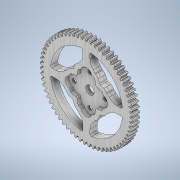
# Autodesk Inventor part: アーム 2段目ギア 大ギア 64
Saved by Autodesk Inventor 2020.2 (Build 242310000, 310)
## iProperties
Created: 2020-05-01
Part Number: アーム 2段目ギア 大ギア 64
Material: アルミニウム 7075
Document SubType Name: Modeling
Designer: mozar
Density: 2.81 g/cm^3
Appearance: サテン - ブラシ仕上げ 重厚
Author: mozar
Autodesk Inventor part; units mm, degrees
(part 1 of 5)
ref_plane "YZ Plane" through (0, 0, 0) normal (1, 0, 0) x (0, 1, 0)
ref_plane "XZ Plane" through (0, 0, 0) normal (0, 1, 0) x (-1, 0, 0)
ref_plane "XY Plane" through (0, 0, 0) normal (0, 0, 1) x (1, 0, 0)
sketch "スケッチ1" plane through (0, 0, 0) normal (0, 0, 1) x (1, 0, 0)
  arc A0 (149.0434, 136.3017) -> (148.894, 135.7475) centre (156.2837, 134.0527) ccw
  arc A1 (149.3046, 137.0392) -> (149.0434, 136.3017) centre (158.5049, 133.3653) ccw
  arc A2 (149.7251, 137.9773) -> (149.3046, 137.0392) centre (160.7701, 132.4624) ccw
  arc A3 (145.9727, 136.2043) -> (145.8783, 135.638) centre (153.3985, 134.6758) ccw
  arc A4 (146.1603, 136.9638) -> (145.9727, 136.2043) centre (155.6764, 134.2093) ccw
  arc A5 (146.4869, 137.9385) -> (146.1603, 136.9638) centre (158.0193, 133.5328) ccw
  arc A6 (142.9263, 135.8063) -> (142.8879, 135.2335) centre (150.4662, 135.013) ccw
  arc A7 (143.0386, 136.5805) -> (142.9263, 135.8063) centre (152.7789, 134.7721) ccw
  arc A8 (143.2681, 137.5826) -> (143.0386, 136.5805) centre (155.1767, 134.3285) ccw
  arc A9 (139.9336, 135.1116) -> (139.9515, 134.5379) centre (147.515, 135.0612) ccw
  arc A10 (139.9695, 135.8932) -> (139.9336, 135.1116) centre (149.8401, 135.0481) ccw
  arc A11 (140.0996, 136.9129) -> (139.9695, 135.8932) centre (152.2699, 134.8417) ccw
  arc A12 (137.0234, 134.127) -> (137.0974, 133.5577) centre (144.5732, 134.8199) ccw
  arc A13 (136.9825, 134.9083) -> (137.0234, 134.127) centre (146.8884, 135.0348) ccw
  arc A14 (137.012, 135.9358) -> (136.9825, 134.9083) centre (149.3267, 135.0675) ccw
  arc A15 (134.2237, 132.8618) -> (134.3532, 132.3026) centre (141.6692, 134.2914) ccw
  arc A16 (134.1064, 133.6353) -> (134.2237, 132.8618) centre (143.9522, 134.7322) ccw
  arc A17 (134.0351, 134.6609) -> (134.1064, 133.6353) centre (146.3756, 135.0037) ccw
  arc A18 (131.5615, 131.3283) -> (131.7452, 130.7845) centre (138.8311, 133.4809) ccw
  arc A19 (131.369, 132.0866) -> (131.5615, 131.3283) centre (141.0599, 134.1433) ccw
  arc A20 (131.1975, 133.1002) -> (131.369, 132.0866) centre (143.445, 134.651) ccw
  arc A21 (129.0624, 129.5413) -> (129.2985, 129.018) centre (136.086, 132.396) ccw
  arc A22 (128.7965, 130.2771) -> (129.0624, 129.5413) centre (138.2392, 133.2737) ccw
  arc A23 (128.5265, 131.269) -> (128.7965, 130.2771) centre (140.563, 134.0128) ccw
  arc A24 (126.7505, 127.5179) -> (127.0368, 127.0203) centre (133.4605, 131.0473) ccw
  arc A25 (126.4138, 128.2241) -> (126.7505, 127.5179) centre (135.5173, 132.1318) ccw
  arc A26 (126.0479, 129.1847) -> (126.4138, 128.2241) centre (137.7575, 133.0951) ccw
  arc A27 (124.6481, 125.2777) -> (124.9818, 124.8105) centre (130.9799, 129.4477) ccw
  arc A28 (124.2438, 125.9474) -> (124.6481, 125.2777) centre (132.9204, 130.7286) ccw
  arc A29 (123.7855, 126.8676) -> (124.2438, 125.9474) centre (135.0554, 131.9069) ccw
  arc A30 (122.7754, 122.8421) -> (123.1533, 122.41) centre (128.6679, 127.6127) ccw
  arc A31 (122.3074, 123.469) -> (122.7754, 122.8421) centre (130.4736, 129.0776) ccw
  arc A32 (121.7611, 124.3398) -> (122.3074, 123.469) centre (132.4828, 130.4595) ccw
  arc A33 (121.1505, 120.2348) -> (121.5689, 119.8417) centre (126.547, 125.56) ccw
  arc A34 (120.6232, 120.8128) -> (121.1505, 120.2348) centre (128.2004, 127.1948) ccw
  arc A35 (119.9942, 121.6258) -> (120.6232, 120.8128) centre (130.0645, 128.767) ccw
  arc A36 (119.7889, 117.4807) -> (120.2438, 117.1305) centre (124.6375, 123.3092) ccw
  arc A37 (119.2076, 118.0042) -> (119.7889, 117.4807) centre (126.1226, 125.0982) ccw
  arc A38 (118.5018, 118.7517) -> (119.2076, 118.0042) centre (127.8237, 126.8455) ccw
  arc A39 (118.7038, 114.6064) -> (119.1909, 114.3025) centre (122.9578, 120.8821) ccw
  arc A40 (118.074, 115.0704) -> (118.7038, 114.6064) centre (124.2604, 122.8081) ccw
  arc A41 (117.2984, 115.7452) -> (118.074, 115.0704) centre (125.782, 124.7137) ccw
  arc A42 (117.9057, 111.6396) -> (118.4202, 111.3849) centre (121.524, 118.302) ccw
  arc A43 (117.2334, 112.0397) -> (117.9057, 111.6396) centre (122.6316, 120.3464) ccw
  arc A44 (116.3954, 112.6351) -> (117.2334, 112.0397) centre (123.9591, 122.392) ccw
  arc A45 (117.4022, 108.6089) -> (117.9392, 108.4058) centre (120.3501, 115.5939) ccw
  arc A46 (116.6939, 108.9411) -> (117.4022, 108.6089) centre (121.252, 117.737) ccw
  arc A47 (115.8016, 109.4516) -> (116.6939, 108.9411) centre (122.3726, 119.9028) ccw
  arc A48 (117.1983, 105.5434) -> (117.7525, 105.394) centre (119.4473, 112.7837) ccw
  arc A49 (116.4608, 105.8046) -> (117.1983, 105.5434) centre (120.1347, 115.0049) ccw
  arc A50 (115.5227, 106.2251) -> (116.4608, 105.8046) centre (121.0376, 117.2701) ccw
  arc A51 (117.2957, 102.4727) -> (117.862, 102.3783) centre (118.8242, 109.8985) ccw
  arc A52 (116.5362, 102.6603) -> (117.2957, 102.4727) centre (119.2907, 112.1764) ccw
  arc A53 (115.5615, 102.9869) -> (116.5362, 102.6603) centre (119.9672, 114.5193) ccw
  arc A54 (117.6937, 99.4263) -> (118.2665, 99.3879) centre (118.487, 106.9662) ccw
  arc A55 (116.9195, 99.5386) -> (117.6937, 99.4263) centre (118.7279, 109.2789) ccw
  arc A56 (115.9174, 99.7681) -> (116.9195, 99.5386) centre (119.1715, 111.6767) ccw
  arc A57 (118.3884, 96.4336) -> (118.9621, 96.4515) centre (118.4388, 104.015) ccw
  arc A58 (117.6068, 96.4695) -> (118.3884, 96.4336) centre (118.4519, 106.3401) ccw
  arc A59 (116.5871, 96.5996) -> (117.6068, 96.4695) centre (118.6583, 108.7699) ccw
  arc A60 (119.373, 93.5234) -> (119.9423, 93.5974) centre (118.6801, 101.0732) ccw
  arc A61 (118.5917, 93.4825) -> (119.373, 93.5234) centre (118.4652, 103.3884) ccw
  arc A62 (117.5642, 93.512) -> (118.5917, 93.4825) centre (118.4325, 105.8267) ccw
  arc A63 (120.6382, 90.7237) -> (121.1974, 90.8532) centre (119.2086, 98.1692) ccw
  arc A64 (119.8647, 90.6064) -> (120.6382, 90.7237) centre (118.7678, 100.4522) ccw
  arc A65 (118.8391, 90.5351) -> (119.8647, 90.6064) centre (118.4963, 102.8756) ccw
  arc A66 (122.1717, 88.0615) -> (122.7155, 88.2452) centre (120.0191, 95.3311) ccw
  arc A67 (121.4134, 87.869) -> (122.1717, 88.0615) centre (119.3567, 97.5599) ccw
  arc A68 (120.3998, 87.6975) -> (121.4134, 87.869) centre (118.849, 99.945) ccw
  arc A69 (123.9587, 85.5624) -> (124.482, 85.7985) centre (121.104, 92.586) ccw
  arc A70 (123.2229, 85.2965) -> (123.9587, 85.5624) centre (120.2263, 94.7392) ccw
  arc A71 (122.231, 85.0265) -> (123.2229, 85.2965) centre (119.4872, 97.063) ccw
  arc A72 (125.9821, 83.2505) -> (126.4797, 83.5368) centre (122.4527, 89.9605) ccw
  arc A73 (125.2759, 82.9138) -> (125.9821, 83.2505) centre (121.3682, 92.0173) ccw
  arc A74 (124.3153, 82.5479) -> (125.2759, 82.9138) centre (120.4049, 94.2575) ccw
  arc A75 (128.2223, 81.1481) -> (128.6895, 81.4818) centre (124.0523, 87.4799) ccw
  arc A76 (127.5526, 80.7438) -> (128.2223, 81.1481) centre (122.7714, 89.4204) ccw
  arc A77 (126.6324, 80.2855) -> (127.5526, 80.7438) centre (121.5931, 91.5554) ccw
  arc A78 (130.6579, 79.2754) -> (131.09, 79.6533) centre (125.8873, 85.1679) ccw
  arc A79 (130.031, 78.8074) -> (130.6579, 79.2754) centre (124.4224, 86.9736) ccw
  arc A80 (129.1602, 78.2611) -> (130.031, 78.8074) centre (123.0405, 88.9828) ccw
  arc A81 (133.2652, 77.6505) -> (133.6583, 78.0689) centre (127.94, 83.047) ccw
  arc A82 (132.6872, 77.1232) -> (133.2652, 77.6505) centre (126.3052, 84.7004) ccw
  arc A83 (131.8742, 76.4942) -> (132.6872, 77.1232) centre (124.733, 86.5645) ccw
  arc A84 (136.0193, 76.2889) -> (136.3695, 76.7438) centre (130.1908, 81.1375) ccw
  arc A85 (135.4958, 75.7076) -> (136.0193, 76.2889) centre (128.4018, 82.6226) ccw
  arc A86 (134.7483, 75.0018) -> (135.4958, 75.7076) centre (126.6545, 84.3237) ccw
  arc A87 (138.8936, 75.2038) -> (139.1975, 75.6909) centre (132.6179, 79.4578) ccw
  arc A88 (138.4296, 74.574) -> (138.8936, 75.2038) centre (130.6919, 80.7604) ccw
  arc A89 (137.7548, 73.7984) -> (138.4296, 74.574) centre (128.7863, 82.282) ccw
  arc A90 (141.8604, 74.4057) -> (142.1151, 74.9202) centre (135.198, 78.024) ccw
  arc A91 (141.4603, 73.7334) -> (141.8604, 74.4057) centre (133.1536, 79.1316) ccw
  arc A92 (140.8649, 72.8954) -> (141.4603, 73.7334) centre (131.108, 80.4591) ccw
  arc A93 (144.8911, 73.9022) -> (145.0942, 74.4392) centre (137.9061, 76.8501) ccw
  arc A94 (144.5589, 73.1939) -> (144.8911, 73.9022) centre (135.763, 77.752) ccw
  arc A95 (144.0484, 72.3016) -> (144.5589, 73.1939) centre (133.5972, 78.8726) ccw
  arc A96 (147.9566, 73.6983) -> (148.106, 74.2525) centre (140.7163, 75.9473) ccw
  arc A97 (147.6954, 72.9608) -> (147.9566, 73.6983) centre (138.4951, 76.6347) ccw
  arc A98 (147.2749, 72.0227) -> (147.6954, 72.9608) centre (136.2299, 77.5376) ccw
  arc A99 (151.0273, 73.7957) -> (151.1217, 74.362) centre (143.6015, 75.3242) ccw
  arc A100 (150.8397, 73.0362) -> (151.0273, 73.7957) centre (141.3236, 75.7907) ccw
  arc A101 (150.5131, 72.0615) -> (150.8397, 73.0362) centre (138.9807, 76.4672) ccw
  arc A102 (154.0737, 74.1937) -> (154.1121, 74.7665) centre (146.5338, 74.987) ccw
  arc A103 (153.9614, 73.4195) -> (154.0737, 74.1937) centre (144.2211, 75.2279) ccw
  arc A104 (153.7319, 72.4174) -> (153.9614, 73.4195) centre (141.8233, 75.6715) ccw
  arc A105 (157.0664, 74.8884) -> (157.0485, 75.4621) centre (149.485, 74.9388) ccw
  arc A106 (157.0305, 74.1068) -> (157.0664, 74.8884) centre (147.1599, 74.9519) ccw
  arc A107 (156.9004, 73.0871) -> (157.0305, 74.1068) centre (144.7301, 75.1583) ccw
  arc A108 (159.9766, 75.873) -> (159.9026, 76.4423) centre (152.4268, 75.1801) ccw
  arc A109 (160.0175, 75.0917) -> (159.9766, 75.873) centre (150.1116, 74.9652) ccw
  arc A110 (159.988, 74.0642) -> (160.0175, 75.0917) centre (147.6733, 74.9325) ccw
  arc A111 (162.7763, 77.1382) -> (162.6468, 77.6974) centre (155.3308, 75.7086) ccw
  arc A112 (162.8936, 76.3647) -> (162.7763, 77.1382) centre (153.0478, 75.2678) ccw
  arc A113 (162.9649, 75.3391) -> (162.8936, 76.3647) centre (150.6244, 74.9963) ccw
  arc A114 (165.4385, 78.6717) -> (165.2548, 79.2155) centre (158.1689, 76.5191) ccw
  arc A115 (165.631, 77.9134) -> (165.4385, 78.6717) centre (155.9401, 75.8567) ccw
  arc A116 (165.8025, 76.8998) -> (165.631, 77.9134) centre (153.555, 75.349) ccw
  arc A117 (167.9376, 80.4587) -> (167.7015, 80.982) centre (160.914, 77.604) ccw
  arc A118 (168.2035, 79.7229) -> (167.9376, 80.4587) centre (158.7608, 76.7263) ccw
  arc A119 (168.4735, 78.731) -> (168.2035, 79.7229) centre (156.437, 75.9872) ccw
  arc A120 (170.2495, 82.4821) -> (169.9632, 82.9797) centre (163.5395, 78.9527) ccw
  arc A121 (170.5862, 81.7759) -> (170.2495, 82.4821) centre (161.4827, 77.8682) ccw
  arc A122 (170.9521, 80.8153) -> (170.5862, 81.7759) centre (159.2425, 76.9049) ccw
  arc A123 (172.3519, 84.7223) -> (172.0182, 85.1895) centre (166.0201, 80.5523) ccw
  arc A124 (172.7562, 84.0526) -> (172.3519, 84.7223) centre (164.0796, 79.2714) ccw
  arc A125 (173.2145, 83.1324) -> (172.7562, 84.0526) centre (161.9446, 78.0931) ccw
  arc A126 (174.2246, 87.1579) -> (173.8467, 87.59) centre (168.3321, 82.3873) ccw
  arc A127 (174.6926, 86.531) -> (174.2246, 87.1579) centre (166.5264, 80.9224) ccw
  arc A128 (175.2389, 85.6602) -> (174.6926, 86.531) centre (164.5172, 79.5405) ccw
  arc A129 (175.8495, 89.7652) -> (175.4311, 90.1583) centre (170.453, 84.44) ccw
  arc A130 (176.3768, 89.1872) -> (175.8495, 89.7652) centre (168.7996, 82.8052) ccw
  arc A131 (177.0058, 88.3742) -> (176.3768, 89.1872) centre (166.9355, 81.233) ccw
  arc A132 (177.2111, 92.5193) -> (176.7562, 92.8695) centre (172.3625, 86.6908) ccw
  arc A133 (177.7924, 91.9958) -> (177.2111, 92.5193) centre (170.8774, 84.9018) ccw
  arc A134 (178.4982, 91.2483) -> (177.7924, 91.9958) centre (169.1763, 83.1545) ccw
  arc A135 (178.2962, 95.3936) -> (177.8091, 95.6975) centre (174.0422, 89.1179) ccw
  arc A136 (178.926, 94.9296) -> (178.2962, 95.3936) centre (172.7396, 87.1919) ccw
  arc A137 (179.7016, 94.2548) -> (178.926, 94.9296) centre (171.218, 85.2863) ccw
  arc A138 (179.0943, 98.3604) -> (178.5798, 98.6151) centre (175.476, 91.698) ccw
  arc A139 (179.7666, 97.9603) -> (179.0943, 98.3604) centre (174.3684, 89.6536) ccw
  arc A140 (180.6046, 97.3649) -> (179.7666, 97.9603) centre (173.0409, 87.608) ccw
  arc A141 (179.5978, 101.3911) -> (179.0608, 101.5942) centre (176.6499, 94.4061) ccw
  arc A142 (180.3061, 101.0589) -> (179.5978, 101.3911) centre (175.748, 92.263) ccw
  arc A143 (181.1984, 100.5484) -> (180.3061, 101.0589) centre (174.6274, 90.0972) ccw
  arc A144 (179.8017, 104.4566) -> (179.2475, 104.606) centre (177.5527, 97.2163) ccw
  arc A145 (180.5392, 104.1954) -> (179.8017, 104.4566) centre (176.8653, 94.9951) ccw
  arc A146 (181.4773, 103.7749) -> (180.5392, 104.1954) centre (175.9624, 92.7299) ccw
  arc A147 (179.7043, 107.5273) -> (179.138, 107.6217) centre (178.1758, 100.1015) ccw
  arc A148 (180.4638, 107.3397) -> (179.7043, 107.5273) centre (177.7093, 97.8236) ccw
  arc A149 (181.4385, 107.0131) -> (180.4638, 107.3397) centre (177.0328, 95.4807) ccw
  arc A150 (179.3063, 110.5737) -> (178.7335, 110.6121) centre (178.513, 103.0338) ccw
  arc A151 (180.0805, 110.4614) -> (179.3063, 110.5737) centre (178.2721, 100.7211) ccw
  arc A152 (181.0826, 110.2319) -> (180.0805, 110.4614) centre (177.8285, 98.3233) ccw
  arc A153 (178.6116, 113.5664) -> (178.0379, 113.5485) centre (178.5612, 105.985) ccw
  arc A154 (179.3932, 113.5305) -> (178.6116, 113.5664) centre (178.5481, 103.6599) ccw
  arc A155 (180.4129, 113.4004) -> (179.3932, 113.5305) centre (178.3417, 101.2301) ccw
  arc A156 (177.627, 116.4766) -> (177.0577, 116.4026) centre (178.3199, 108.9268) ccw
  arc A157 (178.4083, 116.5175) -> (177.627, 116.4766) centre (178.5348, 106.6116) ccw
  arc A158 (179.4358, 116.488) -> (178.4083, 116.5175) centre (178.5675, 104.1733) ccw
  arc A159 (176.3618, 119.2763) -> (175.8026, 119.1468) centre (177.7914, 111.8308) ccw
  arc A160 (177.1353, 119.3936) -> (176.3618, 119.2763) centre (178.2322, 109.5478) ccw
  arc A161 (178.1609, 119.4649) -> (177.1353, 119.3936) centre (178.5037, 107.1244) ccw
  arc A162 (174.8283, 121.9385) -> (174.2845, 121.7548) centre (176.9809, 114.6689) ccw
  arc A163 (175.5866, 122.131) -> (174.8283, 121.9385) centre (177.6433, 112.4401) ccw
  arc A164 (176.6002, 122.3025) -> (175.5866, 122.131) centre (178.151, 110.055) ccw
  arc A165 (173.0413, 124.4376) -> (172.518, 124.2015) centre (175.896, 117.414) ccw
  arc A166 (173.7771, 124.7035) -> (173.0413, 124.4376) centre (176.7737, 115.2608) ccw
  arc A167 (174.769, 124.9735) -> (173.7771, 124.7035) centre (177.5128, 112.937) ccw
  arc A168 (171.0179, 126.7495) -> (170.5203, 126.4632) centre (174.5473, 120.0395) ccw
  arc A169 (171.7241, 127.0862) -> (171.0179, 126.7495) centre (175.6318, 117.9827) ccw
  arc A170 (172.6847, 127.4521) -> (171.7241, 127.0862) centre (176.5951, 115.7425) ccw
  arc A171 (168.7777, 128.8519) -> (168.3105, 128.5182) centre (172.9477, 122.5201) ccw
  arc A172 (169.4474, 129.2562) -> (168.7777, 128.8519) centre (174.2286, 120.5796) ccw
  arc A173 (170.3676, 129.7145) -> (169.4474, 129.2562) centre (175.4069, 118.4446) ccw
  arc A174 (166.3421, 130.7246) -> (165.91, 130.3467) centre (171.1127, 124.8321) ccw
  arc A175 (166.969, 131.1926) -> (166.3421, 130.7246) centre (172.5776, 123.0264) ccw
  arc A176 (167.8398, 131.7389) -> (166.969, 131.1926) centre (173.9595, 121.0172) ccw
  arc A177 (163.7348, 132.3495) -> (163.3417, 131.9311) centre (169.06, 126.953) ccw
  arc A178 (164.3128, 132.8768) -> (163.7348, 132.3495) centre (170.6948, 125.2996) ccw
  arc A179 (165.1258, 133.5058) -> (164.3128, 132.8768) centre (172.267, 123.4355) ccw
  arc A180 (160.9807, 133.7111) -> (160.6305, 133.2562) centre (166.8092, 128.8625) ccw
  arc A181 (161.5042, 134.2924) -> (160.9807, 133.7111) centre (168.5982, 127.3774) ccw
  arc A182 (162.2517, 134.9982) -> (161.5042, 134.2924) centre (170.3455, 125.6763) ccw
  arc A183 (158.1064, 134.7962) -> (157.8025, 134.3091) centre (164.3821, 130.5422) ccw
  arc A184 (158.5704, 135.426) -> (158.1064, 134.7962) centre (166.3081, 129.2396) ccw
  arc A185 (159.2452, 136.2016) -> (158.5704, 135.426) centre (168.2137, 127.718) ccw
  arc A186 (155.1396, 135.5943) -> (154.8849, 135.0798) centre (161.802, 131.976) ccw
  arc A187 (155.5397, 136.2666) -> (155.1396, 135.5943) centre (163.8464, 130.8684) ccw
  arc A188 (156.1351, 137.1046) -> (155.5397, 136.2666) centre (165.892, 129.5409) ccw
  arc A189 (152.1089, 136.0978) -> (151.9058, 135.5608) centre (159.0939, 133.1499) ccw
  arc A190 (152.4411, 136.8061) -> (152.1089, 136.0978) centre (161.237, 132.248) ccw
  arc A191 (152.9516, 137.6984) -> (152.4411, 136.8061) centre (163.4028, 131.1274) ccw
  arc A192 (148.106, 135.7475) -> (147.9566, 136.3017) centre (140.7163, 134.0527) ccw
  arc A193 (147.9566, 136.3017) -> (147.6954, 137.0392) centre (138.4951, 133.3653) ccw
  arc A194 (147.6954, 137.0392) -> (147.2749, 137.9773) centre (136.2299, 132.4624) ccw
  arc A195 (145.0942, 135.5608) -> (144.8911, 136.0978) centre (137.9061, 133.1499) ccw
  arc A196 (144.8911, 136.0978) -> (144.5589, 136.8061) centre (135.763, 132.248) ccw
  arc A197 (144.5589, 136.8061) -> (144.0484, 137.6984) centre (133.5972, 131.1274) ccw
  arc A198 (142.1151, 135.0798) -> (141.8604, 135.5943) centre (135.198, 131.976) ccw
  arc A199 (141.8604, 135.5943) -> (141.4603, 136.2666) centre (133.1536, 130.8684) ccw
  arc A200 (141.4603, 136.2666) -> (140.8649, 137.1046) centre (131.108, 129.5409) ccw
  arc A201 (139.1975, 134.3091) -> (138.8936, 134.7962) centre (132.6179, 130.5422) ccw
  arc A202 (138.8936, 134.7962) -> (138.4296, 135.426) centre (130.6919, 129.2396) ccw
  arc A203 (138.4296, 135.426) -> (137.7548, 136.2016) centre (128.7863, 127.718) ccw
  arc A204 (136.3695, 133.2562) -> (136.0193, 133.7111) centre (130.1908, 128.8625) ccw
  arc A205 (136.0193, 133.7111) -> (135.4958, 134.2924) centre (128.4018, 127.3774) ccw
  arc A206 (135.4958, 134.2924) -> (134.7483, 134.9982) centre (126.6545, 125.6763) ccw
  arc A207 (133.6583, 131.9311) -> (133.2652, 132.3495) centre (127.94, 126.953) ccw
  arc A208 (133.2652, 132.3495) -> (132.6872, 132.8768) centre (126.3052, 125.2996) ccw
  arc A209 (132.6872, 132.8768) -> (131.8742, 133.5058) centre (124.733, 123.4355) ccw
  arc A210 (131.09, 130.3467) -> (130.6579, 130.7246) centre (125.8873, 124.8321) ccw
  arc A211 (130.6579, 130.7246) -> (130.031, 131.1926) centre (124.4224, 123.0264) ccw
  arc A212 (130.031, 131.1926) -> (129.1602, 131.7389) centre (123.0405, 121.0172) ccw
  arc A213 (128.6895, 128.5182) -> (128.2223, 128.8519) centre (124.0523, 122.5201) ccw
  arc A214 (128.2223, 128.8519) -> (127.5526, 129.2562) centre (122.7714, 120.5796) ccw
  arc A215 (127.5526, 129.2562) -> (126.6324, 129.7145) centre (121.5931, 118.4446) ccw
  arc A216 (126.4797, 126.4632) -> (125.9821, 126.7495) centre (122.4527, 120.0395) ccw
  arc A217 (125.9821, 126.7495) -> (125.2759, 127.0862) centre (121.3682, 117.9827) ccw
  arc A218 (125.2759, 127.0862) -> (124.3153, 127.4521) centre (120.4049, 115.7425) ccw
  arc A219 (124.482, 124.2015) -> (123.9587, 124.4376) centre (121.104, 117.414) ccw
  arc A220 (123.9587, 124.4376) -> (123.2229, 124.7035) centre (120.2263, 115.2608) ccw
  arc A221 (123.2229, 124.7035) -> (122.231, 124.9735) centre (119.4872, 112.937) ccw
  arc A222 (122.7155, 121.7548) -> (122.1717, 121.9385) centre (120.0191, 114.6689) ccw
  arc A223 (122.1717, 121.9385) -> (121.4134, 122.131) centre (119.3567, 112.4401) ccw
  arc A224 (121.4134, 122.131) -> (120.3998, 122.3025) centre (118.849, 110.055) ccw
  arc A225 (121.1974, 119.1468) -> (120.6382, 119.2763) centre (119.2086, 111.8308) ccw
  arc A226 (120.6382, 119.2763) -> (119.8647, 119.3936) centre (118.7678, 109.5478) ccw
  arc A227 (119.8647, 119.3936) -> (118.8391, 119.4649) centre (118.4963, 107.1244) ccw
  arc A228 (119.9423, 116.4026) -> (119.373, 116.4766) centre (118.6801, 108.9268) ccw
  arc A229 (119.373, 116.4766) -> (118.5917, 116.5175) centre (118.4652, 106.6116) ccw
  arc A230 (118.5917, 116.5175) -> (117.5642, 116.488) centre (118.4325, 104.1733) ccw
  arc A231 (118.9621, 113.5485) -> (118.3884, 113.5664) centre (118.4388, 105.985) ccw
  arc A232 (118.3884, 113.5664) -> (117.6068, 113.5305) centre (118.4519, 103.6599) ccw
  arc A233 (117.6068, 113.5305) -> (116.5871, 113.4004) centre (118.6583, 101.2301) ccw
  arc A234 (118.2665, 110.6121) -> (117.6937, 110.5737) centre (118.487, 103.0338) ccw
  arc A235 (117.6937, 110.5737) -> (116.9195, 110.4614) centre (118.7279, 100.7211) ccw
  arc A236 (116.9195, 110.4614) -> (115.9174, 110.2319) centre (119.1715, 98.3233) ccw
  arc A237 (117.862, 107.6217) -> (117.2957, 107.5273) centre (118.8242, 100.1015) ccw
  arc A238 (117.2957, 107.5273) -> (116.5362, 107.3397) centre (119.2907, 97.8236) ccw
  arc A239 (116.5362, 107.3397) -> (115.5615, 107.0131) centre (119.9672, 95.4807) ccw
  arc A240 (117.7525, 104.606) -> (117.1983, 104.4566) centre (119.4473, 97.2163) ccw
  arc A241 (117.1983, 104.4566) -> (116.4608, 104.1954) centre (120.1347, 94.9951) ccw
  arc A242 (116.4608, 104.1954) -> (115.5227, 103.7749) centre (121.0376, 92.7299) ccw
  arc A243 (117.9392, 101.5942) -> (117.4022, 101.3911) centre (120.3501, 94.4061) ccw
  arc A244 (117.4022, 101.3911) -> (116.6939, 101.0589) centre (121.252, 92.263) ccw
  arc A245 (116.6939, 101.0589) -> (115.8016, 100.5484) centre (122.3726, 90.0972) ccw
  arc A246 (118.4202, 98.6151) -> (117.9057, 98.3604) centre (121.524, 91.698) ccw
  arc A247 (117.9057, 98.3604) -> (117.2334, 97.9603) centre (122.6316, 89.6536) ccw
  arc A248 (117.2334, 97.9603) -> (116.3954, 97.3649) centre (123.9591, 87.608) ccw
  arc A249 (119.1909, 95.6975) -> (118.7038, 95.3936) centre (122.9578, 89.1179) ccw
  arc A250 (118.7038, 95.3936) -> (118.074, 94.9296) centre (124.2604, 87.1919) ccw
  arc A251 (118.074, 94.9296) -> (117.2984, 94.2548) centre (125.782, 85.2863) ccw
  arc A252 (120.2438, 92.8695) -> (119.7889, 92.5193) centre (124.6375, 86.6908) ccw
  arc A253 (119.7889, 92.5193) -> (119.2076, 91.9958) centre (126.1226, 84.9018) ccw
  arc A254 (119.2076, 91.9958) -> (118.5018, 91.2483) centre (127.8237, 83.1545) ccw
  arc A255 (121.5689, 90.1583) -> (121.1505, 89.7652) centre (126.547, 84.44) ccw
  arc A256 (121.1505, 89.7652) -> (120.6232, 89.1872) centre (128.2004, 82.8052) ccw
  arc A257 (120.6232, 89.1872) -> (119.9942, 88.3742) centre (130.0645, 81.233) ccw
  arc A258 (123.1533, 87.59) -> (122.7754, 87.1579) centre (128.6679, 82.3873) ccw
  arc A259 (122.7754, 87.1579) -> (122.3074, 86.531) centre (130.4736, 80.9224) ccw
  arc A260 (122.3074, 86.531) -> (121.7611, 85.6602) centre (132.4828, 79.5405) ccw
  arc A261 (124.9818, 85.1895) -> (124.6481, 84.7223) centre (130.9799, 80.5523) ccw
  arc A262 (124.6481, 84.7223) -> (124.2438, 84.0526) centre (132.9204, 79.2714) ccw
  arc A263 (124.2438, 84.0526) -> (123.7855, 83.1324) centre (135.0554, 78.0931) ccw
  arc A264 (127.0368, 82.9797) -> (126.7505, 82.4821) centre (133.4605, 78.9527) ccw
  arc A265 (126.7505, 82.4821) -> (126.4138, 81.7759) centre (135.5173, 77.8682) ccw
  arc A266 (126.4138, 81.7759) -> (126.0479, 80.8153) centre (137.7575, 76.9049) ccw
  arc A267 (129.2985, 80.982) -> (129.0624, 80.4587) centre (136.086, 77.604) ccw
  arc A268 (129.0624, 80.4587) -> (128.7965, 79.7229) centre (138.2392, 76.7263) ccw
  arc A269 (128.7965, 79.7229) -> (128.5265, 78.731) centre (140.563, 75.9872) ccw
  arc A270 (131.7452, 79.2155) -> (131.5615, 78.6717) centre (138.8311, 76.5191) ccw
  arc A271 (131.5615, 78.6717) -> (131.369, 77.9134) centre (141.0599, 75.8567) ccw
  arc A272 (131.369, 77.9134) -> (131.1975, 76.8998) centre (143.445, 75.349) ccw
  arc A273 (134.3532, 77.6974) -> (134.2237, 77.1382) centre (141.6692, 75.7086) ccw
  arc A274 (134.2237, 77.1382) -> (134.1064, 76.3647) centre (143.9522, 75.2678) ccw
  arc A275 (134.1064, 76.3647) -> (134.0351, 75.3391) centre (146.3756, 74.9963) ccw
  arc A276 (137.0974, 76.4423) -> (137.0234, 75.873) centre (144.5732, 75.1801) ccw
  arc A277 (137.0234, 75.873) -> (136.9825, 75.0917) centre (146.8884, 74.9652) ccw
  arc A278 (136.9825, 75.0917) -> (137.012, 74.0642) centre (149.3267, 74.9325) ccw
  arc A279 (139.9515, 75.4621) -> (139.9336, 74.8884) centre (147.515, 74.9388) ccw
  arc A280 (139.9336, 74.8884) -> (139.9695, 74.1068) centre (149.8401, 74.9519) ccw
  arc A281 (139.9695, 74.1068) -> (140.0996, 73.0871) centre (152.2699, 75.1583) ccw
  arc A282 (142.8879, 74.7665) -> (142.9263, 74.1937) centre (150.4662, 74.987) ccw
  arc A283 (142.9263, 74.1937) -> (143.0386, 73.4195) centre (152.7789, 75.2279) ccw
  arc A284 (143.0386, 73.4195) -> (143.2681, 72.4174) centre (155.1767, 75.6715) ccw
  arc A285 (145.8783, 74.362) -> (145.9727, 73.7957) centre (153.3985, 75.3242) ccw
  arc A286 (145.9727, 73.7957) -> (146.1603, 73.0362) centre (155.6764, 75.7907) ccw
  arc A287 (146.1603, 73.0362) -> (146.4869, 72.0615) centre (158.0193, 76.4672) ccw
  arc A288 (148.894, 74.2525) -> (149.0434, 73.6983) centre (156.2837, 75.9473) ccw
  arc A289 (149.0434, 73.6983) -> (149.3046, 72.9608) centre (158.5049, 76.6347) ccw
  arc A290 (149.3046, 72.9608) -> (149.7251, 72.0227) centre (160.7701, 77.5376) ccw
  arc A291 (151.9058, 74.4392) -> (152.1089, 73.9022) centre (159.0939, 76.8501) ccw
  arc A292 (152.1089, 73.9022) -> (152.4411, 73.1939) centre (161.237, 77.752) ccw
  arc A293 (152.4411, 73.1939) -> (152.9516, 72.3016) centre (163.4028, 78.8726) ccw
  arc A294 (154.8849, 74.9202) -> (155.1396, 74.4057) centre (161.802, 78.024) ccw
  arc A295 (155.1396, 74.4057) -> (155.5397, 73.7334) centre (163.8464, 79.1316) ccw
  arc A296 (155.5397, 73.7334) -> (156.1351, 72.8954) centre (165.892, 80.4591) ccw
  arc A297 (157.8025, 75.6909) -> (158.1064, 75.2038) centre (164.3821, 79.4578) ccw
  arc A298 (158.1064, 75.2038) -> (158.5704, 74.574) centre (166.3081, 80.7604) ccw
  arc A299 (158.5704, 74.574) -> (159.2452, 73.7984) centre (168.2137, 82.282) ccw
  arc A300 (160.6305, 76.7438) -> (160.9807, 76.2889) centre (166.8092, 81.1375) ccw
  arc A301 (160.9807, 76.2889) -> (161.5042, 75.7076) centre (168.5982, 82.6226) ccw
  arc A302 (161.5042, 75.7076) -> (162.2517, 75.0018) centre (170.3455, 84.3237) ccw
  arc A303 (163.3417, 78.0689) -> (163.7348, 77.6505) centre (169.06, 83.047) ccw
  arc A304 (163.7348, 77.6505) -> (164.3128, 77.1232) centre (170.6948, 84.7004) ccw
  arc A305 (164.3128, 77.1232) -> (165.1258, 76.4942) centre (172.267, 86.5645) ccw
  arc A306 (165.91, 79.6533) -> (166.3421, 79.2754) centre (171.1127, 85.1679) ccw
  arc A307 (166.3421, 79.2754) -> (166.969, 78.8074) centre (172.5776, 86.9736) ccw
  arc A308 (166.969, 78.8074) -> (167.8398, 78.2611) centre (173.9595, 88.9828) ccw
  arc A309 (168.3105, 81.4818) -> (168.7777, 81.1481) centre (172.9477, 87.4799) ccw
  arc A310 (168.7777, 81.1481) -> (169.4474, 80.7438) centre (174.2286, 89.4204) ccw
  arc A311 (169.4474, 80.7438) -> (170.3676, 80.2855) centre (175.4069, 91.5554) ccw
  arc A312 (170.5203, 83.5368) -> (171.0179, 83.2505) centre (174.5473, 89.9605) ccw
  arc A313 (171.0179, 83.2505) -> (171.7241, 82.9138) centre (175.6318, 92.0173) ccw
  arc A314 (171.7241, 82.9138) -> (172.6847, 82.5479) centre (176.5951, 94.2575) ccw
  arc A315 (172.518, 85.7985) -> (173.0413, 85.5624) centre (175.896, 92.586) ccw
  arc A316 (173.0413, 85.5624) -> (173.7771, 85.2965) centre (176.7737, 94.7392) ccw
  arc A317 (173.7771, 85.2965) -> (174.769, 85.0265) centre (177.5128, 97.063) ccw
  arc A318 (174.2845, 88.2452) -> (174.8283, 88.0615) centre (176.9809, 95.3311) ccw
  arc A319 (174.8283, 88.0615) -> (175.5866, 87.869) centre (177.6433, 97.5599) ccw
  arc A320 (175.5866, 87.869) -> (176.6002, 87.6975) centre (178.151, 99.945) ccw
  arc A321 (175.8026, 90.8532) -> (176.3618, 90.7237) centre (177.7914, 98.1692) ccw
  arc A322 (176.3618, 90.7237) -> (177.1353, 90.6064) centre (178.2322, 100.4522) ccw
  arc A323 (177.1353, 90.6064) -> (178.1609, 90.5351) centre (178.5037, 102.8756) ccw
  arc A324 (177.0577, 93.5974) -> (177.627, 93.5234) centre (178.3199, 101.0732) ccw
  arc A325 (177.627, 93.5234) -> (178.4083, 93.4825) centre (178.5348, 103.3884) ccw
  arc A326 (178.4083, 93.4825) -> (179.4358, 93.512) centre (178.5675, 105.8267) ccw
  arc A327 (178.0379, 96.4515) -> (178.6116, 96.4336) centre (178.5612, 104.015) ccw
  arc A328 (178.6116, 96.4336) -> (179.3932, 96.4695) centre (178.5481, 106.3401) ccw
  arc A329 (179.3932, 96.4695) -> (180.4129, 96.5996) centre (178.3417, 108.7699) ccw
  arc A330 (178.7335, 99.3879) -> (179.3063, 99.4263) centre (178.513, 106.9662) ccw
  arc A331 (179.3063, 99.4263) -> (180.0805, 99.5386) centre (178.2721, 109.2789) ccw
  arc A332 (180.0805, 99.5386) -> (181.0826, 99.7681) centre (177.8285, 111.6767) ccw
  arc A333 (179.138, 102.3783) -> (179.7043, 102.4727) centre (178.1758, 109.8985) ccw
  arc A334 (179.7043, 102.4727) -> (180.4638, 102.6603) centre (177.7093, 112.1764) ccw
  arc A335 (180.4638, 102.6603) -> (181.4385, 102.9869) centre (177.0328, 114.5193) ccw
  arc A336 (179.2475, 105.394) -> (179.8017, 105.5434) centre (177.5527, 112.7837) ccw
  arc A337 (179.8017, 105.5434) -> (180.5392, 105.8046) centre (176.8653, 115.0049) ccw
  arc A338 (180.5392, 105.8046) -> (181.4773, 106.2251) centre (175.9624, 117.2701) ccw
  arc A339 (179.0608, 108.4058) -> (179.5978, 108.6089) centre (176.6499, 115.5939) ccw
  arc A340 (179.5978, 108.6089) -> (180.3061, 108.9411) centre (175.748, 117.737) ccw
  arc A341 (180.3061, 108.9411) -> (181.1984, 109.4516) centre (174.6274, 119.9028) ccw
  arc A342 (178.5798, 111.3849) -> (179.0943, 111.6396) centre (175.476, 118.302) ccw
  arc A343 (179.0943, 111.6396) -> (179.7666, 112.0397) centre (174.3684, 120.3464) ccw
  arc A344 (179.7666, 112.0397) -> (180.6046, 112.6351) centre (173.0409, 122.392) ccw
  arc A345 (177.8091, 114.3025) -> (178.2962, 114.6064) centre (174.0422, 120.8821) ccw
  arc A346 (178.2962, 114.6064) -> (178.926, 115.0704) centre (172.7396, 122.8081) ccw
  arc A347 (178.926, 115.0704) -> (179.7016, 115.7452) centre (171.218, 124.7137) ccw
  arc A348 (176.7562, 117.1305) -> (177.2111, 117.4807) centre (172.3625, 123.3092) ccw
  arc A349 (177.2111, 117.4807) -> (177.7924, 118.0042) centre (170.8774, 125.0982) ccw
  arc A350 (177.7924, 118.0042) -> (178.4982, 118.7517) centre (169.1763, 126.8455) ccw
  arc A351 (175.4311, 119.8417) -> (175.8495, 120.2348) centre (170.453, 125.56) ccw
  arc A352 (175.8495, 120.2348) -> (176.3768, 120.8128) centre (168.7996, 127.1948) ccw
  arc A353 (176.3768, 120.8128) -> (177.0058, 121.6258) centre (166.9355, 128.767) ccw
  arc A354 (173.8467, 122.41) -> (174.2246, 122.8421) centre (168.3321, 127.6127) ccw
  arc A355 (174.2246, 122.8421) -> (174.6926, 123.469) centre (166.5264, 129.0776) ccw
  arc A356 (174.6926, 123.469) -> (175.2389, 124.3398) centre (164.5172, 130.4595) ccw
  arc A357 (172.0182, 124.8105) -> (172.3519, 125.2777) centre (166.0201, 129.4477) ccw
  arc A358 (172.3519, 125.2777) -> (172.7562, 125.9474) centre (164.0796, 130.7286) ccw
  arc A359 (172.7562, 125.9474) -> (173.2145, 126.8676) centre (161.9446, 131.9069) ccw
  arc A360 (169.9632, 127.0203) -> (170.2495, 127.5179) centre (163.5395, 131.0473) ccw
  arc A361 (170.2495, 127.5179) -> (170.5862, 128.2241) centre (161.4827, 132.1318) ccw
  arc A362 (170.5862, 128.2241) -> (170.9521, 129.1847) centre (159.2425, 133.0951) ccw
  arc A363 (167.7015, 129.018) -> (167.9376, 129.5413) centre (160.914, 132.396) ccw
  arc A364 (167.9376, 129.5413) -> (168.2035, 130.2771) centre (158.7608, 133.2737) ccw
  arc A365 (168.2035, 130.2771) -> (168.4735, 131.269) centre (156.437, 134.0128) ccw
  arc A366 (165.2548, 130.7845) -> (165.4385, 131.3283) centre (158.1689, 133.4809) ccw
  arc A367 (165.4385, 131.3283) -> (165.631, 132.0866) centre (155.9401, 134.1433) ccw
  arc A368 (165.631, 132.0866) -> (165.8025, 133.1002) centre (153.555, 134.651) ccw
  arc A369 (162.6468, 132.3026) -> (162.7763, 132.8618) centre (155.3308, 134.2914) ccw
  arc A370 (162.7763, 132.8618) -> (162.8936, 133.6353) centre (153.0478, 134.7322) ccw
  arc A371 (162.8936, 133.6353) -> (162.9649, 134.6609) centre (150.6244, 135.0037) ccw
  arc A372 (159.9026, 133.5577) -> (159.9766, 134.127) centre (152.4268, 134.8199) ccw
  arc A373 (159.9766, 134.127) -> (160.0175, 134.9083) centre (150.1116, 135.0348) ccw
  arc A374 (160.0175, 134.9083) -> (159.988, 135.9358) centre (147.6733, 135.0675) ccw
  arc A375 (157.0485, 134.5379) -> (157.0664, 135.1116) centre (149.485, 135.0612) ccw
  arc A376 (157.0664, 135.1116) -> (157.0305, 135.8932) centre (147.1599, 135.0481) ccw
  arc A377 (157.0305, 135.8932) -> (156.9004, 136.9129) centre (144.7301, 134.8417) ccw
  arc A378 (154.1121, 135.2335) -> (154.0737, 135.8063) centre (146.5338, 135.013) ccw
  arc A379 (154.0737, 135.8063) -> (153.9614, 136.5805) centre (144.2211, 134.7721) ccw
  arc A380 (153.9614, 136.5805) -> (153.7319, 137.5826) centre (141.8233, 134.3285) ccw
  arc A381 (151.1217, 135.638) -> (151.0273, 136.2043) centre (143.6015, 134.6758) ccw
  arc A382 (151.0273, 136.2043) -> (150.8397, 136.9638) centre (141.3236, 134.2093) ccw
  arc A383 (150.8397, 136.9638) -> (150.5131, 137.9385) centre (138.9807, 133.5328) ccw
  arc A384 (148.894, 135.7475) -> (148.106, 135.7475) centre (148.5, 105) ccw
  arc A385 (145.8783, 135.638) -> (145.0942, 135.5608) centre (148.5, 105) ccw
  arc A386 (142.8879, 135.2335) -> (142.1151, 135.0798) centre (148.5, 105) ccw
  arc A387 (139.9515, 134.5379) -> (139.1975, 134.3091) centre (148.5, 105) ccw
  arc A388 (137.0974, 133.5577) -> (136.3695, 133.2562) centre (148.5, 105) ccw
  arc A389 (134.3532, 132.3026) -> (133.6583, 131.9311) centre (148.5, 105) ccw
  arc A390 (131.7452, 130.7845) -> (131.09, 130.3467) centre (148.5, 105) ccw
  arc A391 (129.2985, 129.018) -> (128.6895, 128.5182) centre (148.5, 105) ccw
  arc A392 (127.0368, 127.0203) -> (126.4797, 126.4632) centre (148.5, 105) ccw
  arc A393 (124.9818, 124.8105) -> (124.482, 124.2015) centre (148.5, 105) ccw
  arc A394 (123.1533, 122.41) -> (122.7155, 121.7548) centre (148.5, 105) ccw
  arc A395 (121.5689, 119.8417) -> (121.1974, 119.1468) centre (148.5, 105) ccw
  arc A396 (120.2438, 117.1305) -> (119.9423, 116.4026) centre (148.5, 105) ccw
  arc A397 (119.1909, 114.3025) -> (118.9621, 113.5485) centre (148.5, 105) ccw
  arc A398 (118.4202, 111.3849) -> (118.2665, 110.6121) centre (148.5, 105) ccw
  arc A399 (117.9392, 108.4058) -> (117.862, 107.6217) centre (148.5, 105) ccw
  arc A400 (117.7525, 105.394) -> (117.7525, 104.606) centre (148.5, 105) ccw
  arc A401 (117.862, 102.3783) -> (117.9392, 101.5942) centre (148.5, 105) ccw
  arc A402 (118.2665, 99.3879) -> (118.4202, 98.6151) centre (148.5, 105) ccw
  arc A403 (118.9621, 96.4515) -> (119.1909, 95.6975) centre (148.5, 105) ccw
  arc A404 (119.9423, 93.5974) -> (120.2438, 92.8695) centre (148.5, 105) ccw
  arc A405 (121.1974, 90.8532) -> (121.5689, 90.1583) centre (148.5, 105) ccw
  arc A406 (122.7155, 88.2452) -> (123.1533, 87.59) centre (148.5, 105) ccw
  arc A407 (124.482, 85.7985) -> (124.9818, 85.1895) centre (148.5, 105) ccw
  arc A408 (126.4797, 83.5368) -> (127.0368, 82.9797) centre (148.5, 105) ccw
  arc A409 (128.6895, 81.4818) -> (129.2985, 80.982) centre (148.5, 105) ccw
  arc A410 (131.09, 79.6533) -> (131.7452, 79.2155) centre (148.5, 105) ccw
  arc A411 (133.6583, 78.0689) -> (134.3532, 77.6974) centre (148.5, 105) ccw
  arc A412 (136.3695, 76.7438) -> (137.0974, 76.4423) centre (148.5, 105) ccw
  arc A413 (139.1975, 75.6909) -> (139.9515, 75.4621) centre (148.5, 105) ccw
  arc A414 (142.1151, 74.9202) -> (142.8879, 74.7665) centre (148.5, 105) ccw
  arc A415 (145.0942, 74.4392) -> (145.8783, 74.362) centre (148.5, 105) ccw
  arc A416 (148.106, 74.2525) -> (148.894, 74.2525) centre (148.5, 105) ccw
  arc A417 (151.1217, 74.362) -> (151.9058, 74.4392) centre (148.5, 105) ccw
  arc A418 (154.1121, 74.7665) -> (154.8849, 74.9202) centre (148.5, 105) ccw
  arc A419 (157.0485, 75.4621) -> (157.8025, 75.6909) centre (148.5, 105) ccw
  arc A420 (159.9026, 76.4423) -> (160.6305, 76.7438) centre (148.5, 105) ccw
  arc A421 (162.6468, 77.6974) -> (163.3417, 78.0689) centre (148.5, 105) ccw
  arc A422 (165.2548, 79.2155) -> (165.91, 79.6533) centre (148.5, 105) ccw
  arc A423 (167.7015, 80.982) -> (168.3105, 81.4818) centre (148.5, 105) ccw
  arc A424 (169.9632, 82.9797) -> (170.5203, 83.5368) centre (148.5, 105) ccw
  arc A425 (172.0182, 85.1895) -> (172.518, 85.7985) centre (148.5, 105) ccw
  arc A426 (173.8467, 87.59) -> (174.2845, 88.2452) centre (148.5, 105) ccw
  arc A427 (175.4311, 90.1583) -> (175.8026, 90.8532) centre (148.5, 105) ccw
  arc A428 (176.7562, 92.8695) -> (177.0577, 93.5974) centre (148.5, 105) ccw
  arc A429 (177.8091, 95.6975) -> (178.0379, 96.4515) centre (148.5, 105) ccw
  arc A430 (178.5798, 98.6151) -> (178.7335, 99.3879) centre (148.5, 105) ccw
  arc A431 (179.0608, 101.5942) -> (179.138, 102.3783) centre (148.5, 105) ccw
  arc A432 (179.2475, 104.606) -> (179.2475, 105.394) centre (148.5, 105) ccw
  arc A433 (179.138, 107.6217) -> (179.0608, 108.4058) centre (148.5, 105) ccw
  arc A434 (178.7335, 110.6121) -> (178.5798, 111.3849) centre (148.5, 105) ccw
  arc A435 (178.0379, 113.5485) -> (177.8091, 114.3025) centre (148.5, 105) ccw
  arc A436 (177.0577, 116.4026) -> (176.7562, 117.1305) centre (148.5, 105) ccw
  arc A437 (175.8026, 119.1468) -> (175.4311, 119.8417) centre (148.5, 105) ccw
  arc A438 (174.2845, 121.7548) -> (173.8467, 122.41) centre (148.5, 105) ccw
  arc A439 (172.518, 124.2015) -> (172.0182, 124.8105) centre (148.5, 105) ccw
  arc A440 (170.5203, 126.4632) -> (169.9632, 127.0203) centre (148.5, 105) ccw
  arc A441 (168.3105, 128.5182) -> (167.7015, 129.018) centre (148.5, 105) ccw
  arc A442 (165.91, 130.3467) -> (165.2548, 130.7845) centre (148.5, 105) ccw
  arc A443 (163.3417, 131.9311) -> (162.6468, 132.3026) centre (148.5, 105) ccw
  arc A444 (160.6305, 133.2562) -> (159.9026, 133.5577) centre (148.5, 105) ccw
  arc A445 (157.8025, 134.3091) -> (157.0485, 134.5379) centre (148.5, 105) ccw
  arc A446 (154.8849, 135.0798) -> (154.1121, 135.2335) centre (148.5, 105) ccw
  arc A447 (151.9058, 135.5608) -> (151.1217, 135.638) centre (148.5, 105) ccw
  arc A448 (147.2749, 137.9773) -> (146.4869, 137.9385) centre (148.5, 105) ccw
  arc A449 (144.0484, 137.6984) -> (143.2681, 137.5826) centre (148.5, 105) ccw
  arc A450 (140.8649, 137.1046) -> (140.0996, 136.9129) centre (148.5, 105) ccw
  arc A451 (137.7548, 136.2016) -> (137.012, 135.9358) centre (148.5, 105) ccw
  arc A452 (134.7483, 134.9982) -> (134.0351, 134.6609) centre (148.5, 105) ccw
  arc A453 (131.8742, 133.5058) -> (131.1975, 133.1002) centre (148.5, 105) ccw
  arc A454 (129.1602, 131.7389) -> (128.5265, 131.269) centre (148.5, 105) ccw
  arc A455 (126.6324, 129.7145) -> (126.0479, 129.1847) centre (148.5, 105) ccw
  arc A456 (124.3153, 127.4521) -> (123.7855, 126.8676) centre (148.5, 105) ccw
  arc A457 (122.231, 124.9735) -> (121.7611, 124.3398) centre (148.5, 105) ccw
  arc A458 (120.3998, 122.3025) -> (119.9942, 121.6258) centre (148.5, 105) ccw
  arc A459 (118.8391, 119.4649) -> (118.5018, 118.7517) centre (148.5, 105) ccw
  arc A460 (117.5642, 116.488) -> (117.2984, 115.7452) centre (148.5, 105) ccw
  arc A461 (116.5871, 113.4004) -> (116.3954, 112.6351) centre (148.5, 105) ccw
  arc A462 (115.9174, 110.2319) -> (115.8016, 109.4516) centre (148.5, 105) ccw
  arc A463 (115.5615, 107.0131) -> (115.5227, 106.2251) centre (148.5, 105) ccw
  arc A464 (115.5227, 103.7749) -> (115.5615, 102.9869) centre (148.5, 105) ccw
  arc A465 (115.8016, 100.5484) -> (115.9174, 99.7681) centre (148.5, 105) ccw
  arc A466 (116.3954, 97.3649) -> (116.5871, 96.5996) centre (148.5, 105) ccw
  arc A467 (117.2984, 94.2548) -> (117.5642, 93.512) centre (148.5, 105) ccw
  arc A468 (118.5018, 91.2483) -> (118.8391, 90.5351) centre (148.5, 105) ccw
  arc A469 (119.9942, 88.3742) -> (120.3998, 87.6975) centre (148.5, 105) ccw
  arc A470 (121.7611, 85.6602) -> (122.231, 85.0265) centre (148.5, 105) ccw
  arc A471 (123.7855, 83.1324) -> (124.3153, 82.5479) centre (148.5, 105) ccw
  arc A472 (126.0479, 80.8153) -> (126.6324, 80.2855) centre (148.5, 105) ccw
  arc A473 (128.5265, 78.731) -> (129.1602, 78.2611) centre (148.5, 105) ccw
  arc A474 (131.1975, 76.8998) -> (131.8742, 76.4942) centre (148.5, 105) ccw
  arc A475 (134.0351, 75.3391) -> (134.7483, 75.0018) centre (148.5, 105) ccw
  arc A476 (137.012, 74.0642) -> (137.7548, 73.7984) centre (148.5, 105) ccw
  arc A477 (140.0996, 73.0871) -> (140.8649, 72.8954) centre (148.5, 105) ccw
  arc A478 (143.2681, 72.4174) -> (144.0484, 72.3016) centre (148.5, 105) ccw
  arc A479 (146.4869, 72.0615) -> (147.2749, 72.0227) centre (148.5, 105) ccw
  arc A480 (149.7251, 72.0227) -> (150.5131, 72.0615) centre (148.5, 105) ccw
  arc A481 (152.9516, 72.3016) -> (153.7319, 72.4174) centre (148.5, 105) ccw
  arc A482 (156.1351, 72.8954) -> (156.9004, 73.0871) centre (148.5, 105) ccw
  arc A483 (159.2452, 73.7984) -> (159.988, 74.0642) centre (148.5, 105) ccw
  arc A484 (162.2517, 75.0018) -> (162.9649, 75.3391) centre (148.5, 105) ccw
  arc A485 (165.1258, 76.4942) -> (165.8025, 76.8998) centre (148.5, 105) ccw
  arc A486 (167.8398, 78.2611) -> (168.4735, 78.731) centre (148.5, 105) ccw
  arc A487 (170.3676, 80.2855) -> (170.9521, 80.8153) centre (148.5, 105) ccw
  arc A488 (172.6847, 82.5479) -> (173.2145, 83.1324) centre (148.5, 105) ccw
  arc A489 (174.769, 85.0265) -> (175.2389, 85.6602) centre (148.5, 105) ccw
  arc A490 (176.6002, 87.6975) -> (177.0058, 88.3742) centre (148.5, 105) ccw
  arc A491 (178.1609, 90.5351) -> (178.4982, 91.2483) centre (148.5, 105) ccw
  arc A492 (179.4358, 93.512) -> (179.7016, 94.2548) centre (148.5, 105) ccw
  arc A493 (180.4129, 96.5996) -> (180.6046, 97.3649) centre (148.5, 105) ccw
  arc A494 (181.0826, 99.7681) -> (181.1984, 100.5484) centre (148.5, 105) ccw
  arc A495 (181.4385, 102.9869) -> (181.4773, 103.7749) centre (148.5, 105) ccw
  arc A496 (181.4773, 106.2251) -> (181.4385, 107.0131) centre (148.5, 105) ccw
  arc A497 (181.1984, 109.4516) -> (181.0826, 110.2319) centre (148.5, 105) ccw
  arc A498 (180.6046, 112.6351) -> (180.4129, 113.4004) centre (148.5, 105) ccw
  arc A499 (179.7016, 115.7452) -> (179.4358, 116.488) centre (148.5, 105) ccw
  arc A500 (178.4982, 118.7517) -> (178.1609, 119.4649) centre (148.5, 105) ccw
  arc A501 (177.0058, 121.6258) -> (176.6002, 122.3025) centre (148.5, 105) ccw
  arc A502 (175.2389, 124.3398) -> (174.769, 124.9735) centre (148.5, 105) ccw
  arc A503 (173.2145, 126.8676) -> (172.6847, 127.4521) centre (148.5, 105) ccw
  arc A504 (170.9521, 129.1847) -> (170.3676, 129.7145) centre (148.5, 105) ccw
  arc A505 (168.4735, 131.269) -> (167.8398, 131.7389) centre (148.5, 105) ccw
  arc A506 (165.8025, 133.1002) -> (165.1258, 133.5058) centre (148.5, 105) ccw
  arc A507 (162.9649, 134.6609) -> (162.2517, 134.9982) centre (148.5, 105) ccw
  arc A508 (159.988, 135.9358) -> (159.2452, 136.2016) centre (148.5, 105) ccw
  arc A509 (156.9004, 136.9129) -> (156.1351, 137.1046) centre (148.5, 105) ccw
  arc A510 (153.7319, 137.5826) -> (152.9516, 137.6984) centre (148.5, 105) ccw
  arc A511 (150.5131, 137.9385) -> (149.7251, 137.9773) centre (148.5, 105) ccw
  line L0 (113.5, 105) -> (183.5, 105)
  line L1 (148.5, 70) -> (148.5, 140)
  line L2 (201.5, 138) -> (271.5, 138)
  line L3 (201.5, 130) -> (271.5, 130)
  line L4 (201.5, 122) -> (271.5, 122)
  line L5 (201.5, 114) -> (271.5, 114)
  line L6 (201.5, 106) -> (271.5, 106)
  line L7 (201.5, 98) -> (271.5, 98)
  line L8 (201.5, 90) -> (271.5, 90)
  line L9 (201.5, 82) -> (271.5, 82)
  line L10 (201.5, 74) -> (271.5, 74)
  line L11 (201.5, 66) -> (271.5, 66)
  line L12 (201.5, 58) -> (271.5, 58)
  line L13 (201.5, 50) -> (271.5, 50)
  line L14 (201.5, 42) -> (271.5, 42)
  line L15 (201.5, 138) -> (201.5, 42)
  line L16 (271.5, 138) -> (271.5, 42)
  line L17 (236.5, 130) -> (236.5, 42)
  point P0 (0, 0)
  point P1 (207.5, 132)
  point P2 (210, 124)
  point P3 (210, 116)
  point P4 (207.5, 108)
  point P5 (210, 100)
  point P6 (205, 92)
  point P7 (207.5, 84)
  point P8 (207.5, 76)
  point P9 (207.5, 68)
  point P10 (210, 60)
  point P11 (210, 52)
  point P12 (207.5, 44)
  point P13 (237.5, 124)
  point P14 (252.5, 116)
  point P15 (253.75, 108)
  point P16 (250, 100)
  point P17 (252.5, 92)
  point P18 (246.25, 84)
  point P19 (252.5, 76)
  point P20 (250, 68)
  point P21 (247.5, 60)
  point P22 (255, 52)
  point P23 (255, 44)
  point P24 (149.5, 153.5)
  point P25 (149.5, 147.5)
  point P26 (165.6875, 153.5)
  point P27 (167.8125, 147.5)
  constraints: 768 point on circle, 384 centre point, 32 end point, 2 horizontal alignment, 2 midpoint, 2 vertical alignment, 1 horizontal, 1 vertical, 1719 other
extrude "押し出し1" add sketch "スケッチ1" against normal blind 5 contours A1 A2 A511 A383 A382 A381 A447 A189 A190 A191 A510 A380 A379 A378 A446 A186 A187 A188 A509 A377 A376 A375 A445 A183 A184 A185 A508 A374 A373 A372 A444 A180 A181 A182 A507 A371 A370 A369 A443 A177 A178 A179 A506 A368 A367 A366 A442 A174 A175 A176 A505 A365 A364 A363 A441 A171 A172 A173 A504 A362 A361 A360 A440 A168 A169 A170 A503 A359 A358 A357 A439 A165 A166 A167 A502 A356 A355 A354 A438 A162 A163 A164 A501 A353 A352 A351 A437 A159 A160 A161 A500 A350 A349 A348 A436 A156 A157 A158 A499 A347 A346 A345 A435 A153 A154 A155 A498 A344 A343 A342 A434 A150 A151 A152 A497 A341 A340 A339 A433 A147 A148 A149 A496 A338 A337 A336 A432 L0 L1 A384 A0 | L1 L0 A400 A48 A49 A50 A463 A239 A238 A237 A399 A45 A46 A47 A462 A236 A235 A234 A398 A42 A43 A44 A461 A233 A232 A231 A397 A39 A40 A41 A460 A230 A229 A228 A396 A36 A37 A38 A459 A227 A226 A225 A395 A33 A34 A35 A458 A224 A223 A222 A394 A30 A31 A32 A457 A221 A220 A219 A393 A27 A28 A29 A456 A218 A217 A216 A392 A24 A25 A26 A455 A215 A214 A213 A391 A21 A22 A23 A454 A212 A211 A210 A390 A18 A19 A20 A453 A209 A208 A207 A389 A15 A16 A17 A452 A206 A205 A204 A388 A12 A13 A14 A451 A203 A202 A201 A387 A9 A10 A11 A450 A200 A199 A198 A386 A6 A7 A8 A449 A197 A196 A195 A385 A3 A4 A5 A448 A194 A193 A192 A384 | L1 A416 A96 A97 A98 A479 A287 A286 A285 A415 A93 A94 A95 A478 A284 A283 A282 A414 A90 A91 A92 A477 A281 A280 A279 A413 A87 A88 A89 A476 A278 A277 A276 A412 A84 A85 A86 A475 A275 A274 A273 A411 A81 A82 A83 A474 A272 A271 A270 A410 A78 A79 A80 A473 A269 A268 A267 A409 A75 A76 A77 A472 A266 A265 A264 A408 A72 A73 A74 A471 A263 A262 A261 A407 A69 A70 A71 A470 A260 A259 A258 A406 A66 A67 A68 A469 A257 A256 A255 A405 A63 A64 A65 A468 A254 A253 A252 A404 A60 A61 A62 A467 A251 A250 A249 A403 A57 A58 A59 A466 A248 A247 A246 A402 A54 A55 A56 A465 A245 A244 A243 A401 A51 A52 A53 A464 A242 A241 A240 A400 L0 | L0 A432 A144 A145 A146 A495 A335 A334 A333 A431 A141 A142 A143 A494 A332 A331 A330 A430 A138 A139 A140 A493 A329 A328 A327 A429 A135 A136 A137 A492 A326 A325 A324 A428 A132 A133 A134 A491 A323 A322 A321 A427 A129 A130 A131 A490 A320 A319 A318 A426 A126 A127 A128 A489 A317 A316 A315 A425 A123 A124 A125 A488 A314 A313 A312 A424 A120 A121 A122 A487 A311 A310 A309 A423 A117 A118 A119 A486 A308 A307 A306 A422 A114 A115 A116 A485 A305 A304 A303 A421 A111 A112 A113 A484 A302 A301 A300 A420 A108 A109 A110 A483 A299 A298 A297 A419 A105 A106 A107 A482 A296 A295 A294 A418 A102 A103 A104 A481 A293 A292 A291 A417 A99 A100 A101 A480 A290 A289 A288 A416 L1